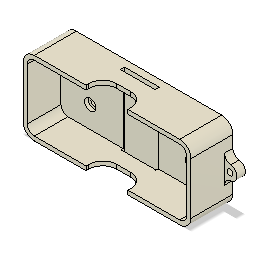
battery_holder (Autodesk Fusion 360 design; units mm, degrees)
Autodesk Fusion 360 part; units mm, degrees
sketch "Sketch1" plane through (0, 0, 0) normal (0, 1, 0) x (1, 0, 0) in component "battery holder"
  line L0 (52, -26.5) -> (-52, -26.5)
  line L1 (-60, -18.5) -> (-60, 18.5)
  line L2 (-52, 26.5) -> (52, 26.5)
  line L3 (60, 18.5) -> (60, -18.5)
  line L4 (60, -26.5) -> (-60, 26.5) construction
  line L5 (-60, -26.5) -> (60, 26.5) construction
  arc A0 (-52, 26.5) -> (-60, 18.5) centre (-52, 18.5) ccw
  arc A1 (-60, -18.5) -> (-52, -26.5) centre (-52, -18.5) ccw
  arc A2 (60, 18.5) -> (52, 26.5) centre (52, 18.5) ccw
  arc A3 (52, -26.5) -> (60, -18.5) centre (52, -18.5) ccw
  circle A4 centre (64, 0) radius 5
  circle A5 centre (-64, 0) radius 5
  line L6 (64, -5) -> (60, -5)
  line L7 (64, 5) -> (60, 5)
  line L8 (-64, -5) -> (-60, -5)
  line L9 (-64, 5) -> (-60, 5)
  circle A6 centre (65, 9.9499) radius 5
  circle A7 centre (65, -9.9499) radius 5
  circle A8 centre (-65, -9.9499) radius 5
  circle A9 centre (-65, 9.9499) radius 5
  circle A10 centre (-36, 8) radius 4
  circle A11 centre (-36, -8) radius 4
  circle A12 centre (36, 8) radius 4
  circle A13 centre (36, -8) radius 4
  point P0 (64, 0)
  point P1 (-64, 0)
  point P2 (-36, 8)
  point P3 (36, 8)
  point P4 (-36, -8)
  point P5 (36, -8)
  dimension "d1_1" = 120
  dimension "d2_1" = 53
  dimension "d3_1" = 8
  dimension "d4_1" = 8
  dimension "d5_1" = 8
  dimension "d6_1" = 8
  dimension "d37_1" = 64
  dimension "d38_1" = 64
  dimension "d39_1" = 10
  dimension "d40_1" = 10
  dimension "d41_1" = 10
  dimension "d42_1" = 10
  dimension "d43_1" = 10
  dimension "d44_1" = 10
  dimension "d52_1" = 8
  dimension "d53_1" = 36
  dimension "d56_1" = 72
  dimension "d57_1" = -16
  dimension "d58_1" = 8
  dimension "d59_1" = 8
  dimension "d60_1" = 8
  dimension "d61_1" = 8
  constraint horizontal L0
  constraint perpendicular L0 L1
  constraint parallel L0 L2
  constraint parallel L1 L3
  constraint coincident L4 origin
  constraint coincident L5 origin
  constraint coincident L4.end L2
  constraint coincident L4.end L1
  constraint tangent L2 A0
  constraint tangent L1 A0
  constraint coincident L5.start L0
  constraint coincident L5.start L1
  constraint tangent L0 A1
  constraint tangent L1 A1
  constraint coincident L5.end L3
  constraint coincident L5.end L2
  constraint tangent L3 A2
  constraint tangent L2 A2
  constraint coincident L4.start L3
  constraint coincident L4.start L0
  constraint tangent L3 A3
  constraint tangent L0 A3
  constraint horizontal origin P0
  constraint horizontal origin P1
  constraint coincident P0 A4.centre
  constraint coincident P1 A5.centre
  constraint coincident A4 L6.start
  constraint coincident L3 L6.end
  constraint tangent A4 L6
  constraint perpendicular L3 L6
  constraint coincident A4 L7.start
  constraint coincident L3 L7.end
  constraint tangent A4 L7
  constraint perpendicular L3 L7
  constraint coincident A5 L8.start
  constraint coincident L1 L8.end
  constraint tangent A5 L8
  constraint perpendicular L1 L8
  constraint coincident A5 L9.start
  constraint coincident L1 L9.end
  constraint tangent A5 L9
  constraint perpendicular L1 L9
  constraint tangent L3 A6
  constraint tangent A4 A6
  constraint tangent L3 A7
  constraint tangent A4 A7
  constraint tangent A5 A8
  constraint tangent L1 A8
  constraint tangent A5 A9
  constraint tangent L1 A9
  constraint coincident P2 A10.centre
  constraint coincident P4 A11.centre
  constraint coincident P3 A12.centre
  constraint coincident P5 A13.centre
  measures "d1_1" distance of L4.end L5.end
  measures "d2_1" distance of L5.start L4.end
  measures "d3_1" radius of A0
  measures "d4_1" radius of A1
  measures "d5_1" radius of A2
  measures "d6_1" radius of A3
  measures "d37_1" distance of origin A4.centre
  measures "d38_1" distance of origin P1
  measures "d39_1" diameter of A4
  measures "d40_1" diameter of A5
  measures "d41_1" diameter of A6
  measures "d42_1" diameter of A7
  measures "d43_1" diameter of A8
  measures "d44_1" diameter of A9
  measures "d52_1" vertical distance of origin P2
  measures "d53_1" horizontal distance of origin P2
  measures "d58_1" diameter of A10
  measures "d59_1" diameter of A11
  measures "d60_1" diameter of A12
  measures "d61_1" diameter of A13
extrude "Extrude1" add sketch "Sketch1" along normal blind 6 contours L0 L1 L2 L3 A0 A1 A2 A3 A4 A5 | L3 A4 | L1 A5 picked at (59.8711, 0.7998) picked at (-59.672, 0.807) in component "battery holder"
extrude "Extrude2" add sketch "Sketch1" along normal blind 30 thin wall 3 on the right open curves A1 L1 A0 L2 A2 L3 A3 L0 in component "battery holder"
sketch "Sketch2" plane through (0, 0, 26.5) normal (0, 0, 1) x (1, 0, 0) in component "battery holder"
  line L0 (-52, 0) -> (52, 0)
  line L1 (52, 0) -> (52, 30)
  line L2 (52, 30) -> (-52, 30)
  line L3 (-52, 30) -> (-52, 0)
  line L4 (5, 18) -> (-5, 18)
  line L5 (-15, 28) -> (-15, 38)
  line L6 (-15, 38) -> (15, 38)
  line L7 (15, 38) -> (15, 28)
  line L8 (15, 18) -> (-15, 38) construction
  line L9 (-15, 18) -> (15, 38) construction
  arc A0 (-15, 28) -> (-5, 18) centre (-5, 28) ccw
  arc A1 (5, 18) -> (15, 28) centre (5, 28) ccw
  point P0 (0, 28)
  dimension "d27_1" = 30
  dimension "d28_1" = 20
  dimension "d29_1" = 18
  dimension "d50_1" = 10
  dimension "d51_1" = 10
  constraint horizontal L4
  constraint perpendicular L4 L5
  constraint parallel L4 L6
  constraint parallel L5 L7
  constraint coincident L8 P0
  constraint coincident L9 P0
  constraint vertical origin P0
  constraint coincident L9.start L5
  constraint coincident L9.start L4
  constraint tangent L5 A0
  constraint tangent L4 A0
  constraint coincident L8.start L4
  constraint coincident L8.start L7
  constraint tangent L4 A1
  constraint tangent L7 A1
  measures "d27_1" distance of L5.end L6.end
  measures "d28_1" distance of L9.start L5.end
  measures "d29_1" vertical distance of origin L8.start
  measures "d50_1" radius of A0
  measures "d51_1" radius of A1
extrude "Extrude4" cut sketch "Sketch2" against normal blind 60 contours L2 L4 L5 L7 A0 A1 in component "battery holder"
sketch "Sketch3" plane through (0, 0, 26.5) normal (0, 0, 1) x (1, 0, 0) in component "battery holder"
  line L0 (15, 30) -> (15, 28)
  line L1 (5, 18) -> (-5, 18)
  line L2 (-15, 28) -> (-15, 30)
  line L3 (-15, 30) -> (-52, 30)
  line L4 (-52, 30) -> (-52, 0)
  line L5 (-52, 0) -> (52, 0)
  line L6 (52, 0) -> (52, 30)
  line L7 (52, 30) -> (15, 30)
  line L8 (12.5, 5) -> (-12.5, 5)
  line L9 (-12.5, 5) -> (-12.5, 7.5)
  line L10 (-12.5, 7.5) -> (12.5, 7.5)
  line L11 (12.5, 7.5) -> (12.5, 5)
  line L12 (12.5, 5) -> (-12.5, 7.5) construction
  line L13 (-12.5, 5) -> (12.5, 7.5) construction
  arc A0 (5, 18) -> (15, 28) centre (5, 28) ccw
  arc A1 (-15, 28) -> (-5, 18) centre (-5, 28) ccw
  point P0 (0, 6.25)
  dimension "d32_1" = 25
  dimension "d33_1" = 2.5
  dimension "d34_1" = 5
  constraint horizontal L8
  constraint perpendicular L8 L9
  constraint parallel L8 L10
  constraint parallel L9 L11
  constraint coincident L12 P0
  constraint coincident L13 P0
  constraint vertical origin P0
  measures "d32_1" distance of L9.end L10.end
  measures "d33_1" distance of L8.end L9.end
  measures "d34_1" vertical distance of origin L8.start
extrude "Extrude5" cut sketch "Sketch3" against normal blind 60 contours L8 L9 L10 L11 in component "battery holder"
extrude "Extrude6" add sketch "Sketch1" along normal blind 6 contours L3 A4 L6 A7 | L1 A5 L8 A8 | L3 A4 L6 | L3 A4 | L1 A5 L8 | L1 A5 | L3 A4 | L1 A5 | L1 A5 L9 A9 | L3 A4 L7 | L3 A4 L7 A6 | L1 A5 L9 in component "battery holder"
hole "Hole1" at (64, 0, 0) at (-64, 0, 0) direction (0, 1, 0) diameter 4.2 depth 6 tip angle 118 in component "battery holder"
extrude "Extrude7" add sketch "Sketch1" along normal blind 3.4 contours A10 | A11 | A12 | A13 in component "battery holder"
hole "Hole2" at (-36, 0, -8) at (-36, 0, 8) at (36, 0, -8) at (36, 0, 8) direction (0, 1, 0) diameter 4.2 depth 4 tip angle 118 in component "battery holder"
chamfer "Chamfer1" distance 0.5 angle 45 2 edges at (0, 7.5, 26.5) (0, 7.5, -26.5) in component "battery holder"
move_body "Move1" bodies 1 to x (1, 0, 0) y (0, 0, 1) z (0, -1, 0) at (0, -26.5, -26.5) in component "battery holder"
component "battery holder" placed x (1, 0, 0) y (0, 1, 0) z (0, 0, 1) at (0, 0, 0)
